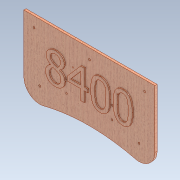
# Autodesk Inventor part: FTC Outside Panels
Saved by Autodesk Inventor 2020 (Build 240168000, 168)
## iProperties
Created: 2022-09-23
Part Number: FTC Outside Panels
Material: Wood (Oak)
Document SubType Name: Modeling
Designer: Jason
Density: 0.76 g/cm^3
Appearance: White Oak - Natural Medium Gloss
Mass: 371.39 g
Surface Area: 1832.51 cm^2
Volume: 488.671 cm^3
Author: Allan
Autodesk Inventor part; units mm, degrees
ref_plane "YZ Plane" through (0, 0, 0) normal (1, 0, 0) x (0, 1, 0)
ref_plane "XZ Plane" through (0, 0, 0) normal (0, 1, 0) x (-1, 0, 0)
ref_plane "XY Plane" through (0, 0, 0) normal (0, 0, 1) x (1, 0, 0)
sketch "Sketch1" plane through (0, 0, 0) normal (0, 0, 1) x (1, 0, 0)
  line L0 (40.3696, 0) -> (44.816, 0)
  line L1 (293.0054, 0) -> (287.9217, 0)
  arc A0 (0, 40.3696) -> (53.3921, 2.1581) centre (40.3696, 40.3696) ccw
  arc A1 (283.1915, 1.211) -> (333.375, 40.3696) centre (293.0054, 40.3696) ccw
  arc A2 (166.6875, 15.627) -> (44.816, 0) centre (166.3688, -464.9274) ccw
  arc A3 (287.9217, 0) -> (283.1915, 1.211) centre (166.3688, -464.9274) ccw
  arc A4 (53.3921, 2.1581) -> (44.816, 0) centre (166.3688, -464.9274) ccw
  arc A5 (287.9217, 0) -> (166.6875, 15.627) centre (166.3688, -464.9274) ccw
  line L2 (0, 40.3696) -> (0, 187.5234)
  line L3 (333.375, 187.5234) -> (333.375, 40.3696)
  line L4 (0, 187.5234) -> (333.375, 187.5234)
  point P0 (0, 0)
  point P1 (46.8129, 0.5175)
  dimension "d69" = 333.375
  constraints: 16 point on circle, 10 end point, 6 centre point, 1 perpendicular, 1 vertical
  measures "d69" distance between parallel lines of L3 L2
extrude "Extrusion1" add sketch "Sketch1" along normal blind 5.5563 contours A0 L2 L4 L3 A1 A5 A2
sketch "Sketch5" plane through (0, 0, 5.5563) normal (0, 0, 1) x (1, 0, 0)
  line L0 (53.8343, 140.6282) -> (283.9977, 140.6282) construction
  line L1 (283.9977, 140.6282) -> (283.9977, 59.079) construction
  line L2 (283.9977, 59.079) -> (53.8343, 59.079) construction
  line L3 (53.8343, 59.079) -> (53.8343, 140.6282) construction
  spline S0 degree 2 poles (82.4247, 60.9702) (76.7437, 60.9702) (67.4193, 64.3665) (64.1466, 67.5157) knots 0 0 0 1 2 2 2
  spline S1 degree 2 poles (64.1466, 67.5157) (60.9355, 70.6033) (57.601, 79.0013) (57.601, 83.7561) knots 0 0 0 1 2 2 2
  spline S2 degree 2 poles (57.601, 83.7561) (57.601, 89.9311) (64.2083, 100.3052) (70.5069, 103.3927) knots 0 0 0 1 2 2 2
  line L4 (70.5069, 103.3927) -> (70.5069, 103.7015)
  spline S3 degree 2 poles (70.5069, 103.7015) (64.8876, 106.9743) (59.4535, 114.7548) (59.4535, 120.5593) knots 0 0 0 1 2 2 2
  spline S4 degree 2 poles (59.4535, 120.5593) (59.4535, 129.1426) (72.4211, 140.6282) (82.4247, 140.6282) knots 0 0 0 1 2 2 2
  spline S5 degree 2 poles (82.4247, 140.6282) (92.7988, 140.6282) (105.3341, 129.7602) (105.3341, 121.2386) knots 0 0 0 1 2 2 2
  spline S6 degree 2 poles (105.3341, 121.2386) (105.3341, 116.1133) (99.3443, 106.1097) (93.725, 103.2692) knots 0 0 0 1 2 2 2
  line L5 (93.725, 103.2692) -> (93.725, 102.9605)
  spline S7 degree 2 poles (93.725, 102.9605) (100.3941, 99.873) (107.2484, 90.9809) (107.2484, 83.9414) knots 0 0 0 1 2 2 2
  spline S8 degree 2 poles (107.2484, 83.9414) (107.2484, 74.1848) (93.0458, 60.9702) (82.4247, 60.9702) knots 0 0 0 1 2 2 2
  spline S9 degree 2 poles (96.7508, 82.9533) (96.7508, 87.6464) (93.0458, 93.2039) (87.797, 96.0444) knots 0 0 0 1 2 2 2
  spline S10 degree 2 poles (87.797, 96.0444) (86.068, 97.0324) (80.2634, 99.3172) (76.6202, 100.7992) knots 0 0 0 1 2 2 2
  spline S11 degree 2 poles (76.6202, 100.7992) (72.4211, 98.0204) (67.9133, 89.7459) (67.9133, 84.4971) knots 0 0 0 1 2 2 2
  spline S12 degree 2 poles (67.9133, 84.4971) (67.9133, 77.5811) (76.2496, 68.5655) (82.5482, 68.5655) knots 0 0 0 1 2 2 2
  spline S13 degree 2 poles (82.5482, 68.5655) (88.9702, 68.5655) (96.7508, 76.2843) (96.7508, 82.9533) knots 0 0 0 1 2 2 2
  spline S14 degree 2 poles (95.3305, 121.1151) (95.3305, 126.2404) (88.4762, 133.0947) (82.3629, 133.0947) knots 0 0 0 1 2 2 2
  spline S15 degree 2 poles (82.3629, 133.0947) (76.8054, 133.0947) (69.7041, 126.9814) (69.7041, 121.7326) knots 0 0 0 1 2 2 2
  spline S16 degree 2 poles (69.7041, 121.7326) (69.7041, 117.9658) (73.3474, 112.717) (76.9907, 110.6175) knots 0 0 0 1 2 2 2
  spline S17 degree 2 poles (76.9907, 110.6175) (78.5344, 109.753) (85.08, 106.7273) (87.7352, 105.8627) knots 0 0 0 1 2 2 2
  spline S18 degree 2 poles (87.7352, 105.8627) (92.1813, 109.259) (95.3305, 116.4838) (95.3305, 121.1151) knots 0 0 0 1 2 2 2
  line L6 (165.6025, 88.8814) -> (156.5252, 88.8814)
  line L7 (156.5252, 88.8814) -> (156.5252, 62.6992)
  line L8 (156.5252, 62.6992) -> (146.7069, 62.6992)
  line L9 (146.7069, 62.6992) -> (146.7069, 88.8814)
  line L10 (146.7069, 88.8814) -> (113.0529, 88.8814)
  line L11 (113.0529, 88.8814) -> (113.0529, 99.626)
  line L12 (113.0529, 99.626) -> (147.1391, 138.8992)
  line L13 (147.1391, 138.8992) -> (156.5252, 138.8992)
  line L14 (156.5252, 138.8992) -> (156.5252, 97.0942)
  line L15 (156.5252, 97.0942) -> (165.6025, 97.0942)
  line L16 (165.6025, 97.0942) -> (165.6025, 88.8814)
  line L17 (146.7069, 97.0942) -> (146.7069, 126.8579)
  line L18 (146.7069, 126.8579) -> (121.0804, 97.0942)
  line L19 (121.0804, 97.0942) -> (146.7069, 97.0942)
  spline S19 degree 2 poles (221.1778, 100.7992) (221.1778, 80.2981) (209.26, 61.0937) (196.8482, 61.0937) knots 0 0 0 1 2 2 2
  spline S20 degree 2 poles (196.8482, 61.0937) (184.2511, 61.0937) (172.4568, 80.6686) (172.4568, 100.7375) knots 0 0 0 1 2 2 2
  spline S21 degree 2 poles (172.4568, 100.7375) (172.4568, 121.3621) (184.3746, 140.443) (196.8482, 140.443) knots 0 0 0 1 2 2 2
  spline S22 degree 2 poles (196.8482, 140.443) (209.3835, 140.443) (221.1778, 120.6828) (221.1778, 100.7992) knots 0 0 0 1 2 2 2
  spline S23 degree 2 poles (208.0868, 77.5811) (209.5688, 81.3478) (210.8038, 92.9569) (210.8038, 100.7992) knots 0 0 0 1 2 2 2
  spline S24 degree 2 poles (210.8038, 100.7992) (210.8038, 108.6415) (209.5688, 120.1888) (208.025, 124.0791) knots 0 0 0 1 2 2 2
  spline S25 degree 2 poles (208.025, 124.0791) (206.4813, 127.9694) (201.109, 131.9832) (196.8482, 131.9832) knots 0 0 0 1 2 2 2
  spline S26 degree 2 poles (196.8482, 131.9832) (192.5874, 131.9832) (187.0916, 127.9694) (185.4861, 123.9556) knots 0 0 0 1 2 2 2
  spline S27 degree 2 poles (185.4861, 123.9556) (183.9424, 120.0653) (182.8308, 108.2093) (182.8308, 100.7375) knots 0 0 0 1 2 2 2
  spline S28 degree 2 poles (182.8308, 100.7375) (182.8308, 92.7099) (183.8189, 81.9653) (185.4244, 77.7663) knots 0 0 0 1 2 2 2
  spline S29 degree 2 poles (185.4244, 77.7663) (186.9064, 73.8143) (192.4022, 69.5535) (196.8482, 69.5535) knots 0 0 0 1 2 2 2
  spline S30 degree 2 poles (196.8482, 69.5535) (201.0472, 69.5535) (206.543, 73.5673) (208.0868, 77.5811) knots 0 0 0 1 2 2 2
  spline S31 degree 2 poles (278.3587, 100.7992) (278.3587, 80.2981) (266.4409, 61.0937) (254.0291, 61.0937) knots 0 0 0 1 2 2 2
  spline S32 degree 2 poles (254.0291, 61.0937) (241.432, 61.0937) (229.6377, 80.6686) (229.6377, 100.7375) knots 0 0 0 1 2 2 2
  spline S33 degree 2 poles (229.6377, 100.7375) (229.6377, 121.3621) (241.5555, 140.443) (254.0291, 140.443) knots 0 0 0 1 2 2 2
  spline S34 degree 2 poles (254.0291, 140.443) (266.5644, 140.443) (278.3587, 120.6828) (278.3587, 100.7992) knots 0 0 0 1 2 2 2
  spline S35 degree 2 poles (265.2676, 77.5811) (266.7496, 81.3478) (267.9847, 92.9569) (267.9847, 100.7992) knots 0 0 0 1 2 2 2
  spline S36 degree 2 poles (267.9847, 100.7992) (267.9847, 108.6415) (266.7496, 120.1888) (265.2059, 124.0791) knots 0 0 0 1 2 2 2
  spline S37 degree 2 poles (265.2059, 124.0791) (263.6621, 127.9694) (258.2898, 131.9832) (254.0291, 131.9832) knots 0 0 0 1 2 2 2
  spline S38 degree 2 poles (254.0291, 131.9832) (249.7683, 131.9832) (244.2725, 127.9694) (242.667, 123.9556) knots 0 0 0 1 2 2 2
  spline S39 degree 2 poles (242.667, 123.9556) (241.1232, 120.0653) (240.0117, 108.2093) (240.0117, 100.7375) knots 0 0 0 1 2 2 2
  spline S40 degree 2 poles (240.0117, 100.7375) (240.0117, 92.7099) (240.9997, 81.9653) (242.6052, 77.7663) knots 0 0 0 1 2 2 2
  spline S41 degree 2 poles (242.6052, 77.7663) (244.0872, 73.8143) (249.583, 69.5535) (254.0291, 69.5535) knots 0 0 0 1 2 2 2
  spline S42 degree 2 poles (254.0291, 69.5535) (258.2281, 69.5535) (263.7239, 73.5673) (265.2676, 77.5811) knots 0 0 0 1 2 2 2
  point P0 (0, 0)
  constraints: 2 other
sketch "Sketch6" plane through (0, 0, 5.5563) normal (0, 0, 1) x (1, 0, 0)
  line L0 (333.375, 187.5234) -> (0, 187.5234)
  line L1 (0, 187.5234) -> (0, 40.3696)
  circle A0 centre (26.0449, 161.4785) radius 2.4066
  line L2 (333.375, 40.3696) -> (333.375, 187.5234)
  circle A1 centre (307.3301, 161.4785) radius 2.4066
  circle A2 centre (166.6875, 161.4785) radius 2.4066
  arc A3 (283.1915, 1.211) -> (333.375, 40.3696) centre (293.0054, 40.3696) ccw
  circle A4 centre (293.0054, 40.3696) radius 2.4066
  arc A5 (0, 40.3696) -> (46.8129, 0.5175) centre (40.3696, 40.3696) ccw
  circle A6 centre (40.3696, 40.3696) radius 2.4066
  point P0 (0, 0)
  point P1 (0, 0)
  dimension "d70" = 333.375
  constraints: 7 centre point, 6 end point, 4 point on circle
  measures "d70" distance between parallel lines of L2 L1
extrude "Extrusion6" cut sketch "Sketch6" against normal up to surface (5.5563 mm away)
sketch "Sketch7" plane through (0, 0, 5.5563) normal (0, 0, 1) x (1, 0, 0)
  ellipse E0 centre (224.6285, 89.9888) end of major axis (224.6247, 91.9888) minor radius 2
  ellipse E1 centre (224.6285, 57.9868) end of major axis (224.6212, 59.9867) minor radius 2
  circle A0 centre (292.998, 40.3696) radius 2.9337
  line L0 (292.998, 40.3696) -> (224.6211, 40.3696)
  line L1 (224.6285, 40.3696) -> (224.6285, 57.9868)
  ellipse E2 centre (108.7466, 89.9867) end of major axis (108.7427, 91.9867) minor radius 2
  ellipse E3 centre (108.7466, 57.9868) end of major axis (108.7392, 59.9867) minor radius 2
  line L2 (108.7466, 40.3696) -> (108.7466, 57.9868)
  circle A1 centre (224.6594, 73.9878) radius 4.699
  circle A2 centre (108.7774, 73.9878) radius 4.699
  circle A3 centre (40.3696, 40.3696) radius 2.9337
  line L3 (40.3696, 40.3696) -> (108.7466, 40.3696)
  circle A4 centre (40.3696, 40.3696) radius 2.4066 projected
  circle A5 centre (293.0054, 40.3696) radius 2.4066 projected
  line L4 (40.3696, 40.3696) -> (293.0054, 40.3696)
  line L5 (224.6285, 89.9888) -> (224.6285, 57.9868)
  line L6 (108.7466, 89.9867) -> (108.7466, 57.9868)
  point P0 (0, 0)
  point P1 (0, 0)
  point P2 (166.6979, 70.2541)
  dimension "d59" = 17.6171
  dimension "d60" = 68.3769
  dimension "d61" = 17.6171
  dimension "d62" = 9.398
  dimension "d63" = 9.398
  dimension "d64" = 68.3769
  dimension "d71" = 252.6357
  dimension "d72" = 252.6284
  constraints: 14 end point, 4 centre point, 3 horizontal, 3 vertical, 1 coincident, 1 perpendicular, 8 other
  measures "d59" distance of L1.start L1.end
  measures "d60" distance of L0.end L0.start
  measures "d61" distance of L2.start L2.end
  measures "d62" diameter of A1
  measures "d63" diameter of A2
  measures "d64" distance of L3.end L3.start
  measures "d71" distance of L4.start L4.end
  measures "d72" distance of L0.start L3.start
extrude "Extrusion7" cut sketch "Sketch7" against normal through all contours E0 | E1 L5 L1 | L1 L5 E1 | E2 | E3 L6 L2 | L2 L6 E3
sketch "Sketch8" plane through (0, 0, 5.5563) normal (0, 0, 1) x (1, 0, 0)
  ellipse E0 centre (240.6029, 123.3584) end of major axis (240.6055, 122.0058) minor radius 1.3525
  ellipse E1 centre (208.6031, 123.2969) end of major axis (208.6057, 121.9443) minor radius 1.3525
  ellipse E2 centre (224.6285, 89.9888) end of major axis (224.6247, 91.9888) minor radius 2
  ellipse E3 centre (224.6285, 89.9888) end of major axis (224.6247, 91.9888) minor radius 2 projected
  ellipse E4 centre (124.721, 123.3562) end of major axis (124.7236, 122.0037) minor radius 1.3525
  ellipse E5 centre (92.7211, 123.2947) end of major axis (92.7237, 121.9422) minor radius 1.3525
  ellipse E6 centre (108.7466, 89.9867) end of major axis (108.7427, 91.9867) minor radius 2
  ellipse E7 centre (108.7466, 89.9867) end of major axis (108.7427, 91.9867) minor radius 2 projected
  point P0 (0, 0)
  constraints: 4 centre point, 6 other
extrude "Extrusion8" cut sketch "Sketch8" against normal through all contours E0 | E1 | E4 | E5
emboss "Emboss1" sketch "Sketch5" operation add depth 2.54 direction (0, 0, -1)
body "Solid1"
